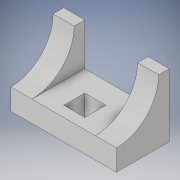
# Autodesk Inventor part: Part2
Saved by Autodesk Inventor 2017 (Build 210142000, 142)
## iProperties
Created: 2016-11-01
Part Number: Part2
Material: Generic
Document SubType Name: Modeling
Designer: s411888
Density: 1 g/cm^3
Appearance: Default
Author: s411888
Autodesk Inventor part; units mm, degrees
ref_plane "YZ Plane" through (0, 0, 0) normal (1, 0, 0) x (0, 1, 0)
ref_plane "XZ Plane" through (0, 0, 0) normal (0, 1, 0) x (-1, 0, 0)
ref_plane "XY Plane" through (0, 0, 0) normal (0, 0, 1) x (1, 0, 0)
sketch "Sketch1" plane through (0, 0, 0) normal (0, 1, 0) x (-1, 0, 0)
  line L0 (35.0198, 16.1328) -> (-28.4802, 16.1328)
  line L1 (-28.4802, 16.1328) -> (-28.4802, -15.6172)
  line L2 (-28.4802, -15.6172) -> (35.0198, -15.6172)
  line L3 (35.0198, -15.6172) -> (35.0198, 16.1328)
  point P0 (0, 0)
  dimension "d0" = 63.5
  dimension "d1" = 31.75
  constraints: 8 end point, 2 parallel, 1 horizontal, 1 perpendicular
  measures "d0" distance of L2.end L1.end
  measures "d1" distance of L0.end L1.end
extrude "Extrusion1" add sketch "Sketch1" along normal blind 38.1
sketch "Sketch2" plane through (0, 38.1, 0) normal (0, 1, 0) x (1, 0, 0)
  line L0 (28.4802, -16.1328) -> (28.4802, 15.6172) projected
  line L1 (15.7802, 15.6172) -> (15.7802, 9.2672)
  line L2 (28.4802, 9.2672) -> (28.4802, 15.6172)
  line L3 (15.7802, 15.6172) -> (-22.3198, 15.6172)
  line L4 (-22.3198, 15.6172) -> (-22.3198, -16.1328)
  line L5 (-22.3198, -16.1328) -> (15.7802, -16.1328)
  line L6 (15.7802, -16.1328) -> (15.7802, 15.6172)
  point P0 (0, 0)
  dimension "d4" = 12.7
  dimension "d5" = 6.35
  dimension "d6" = 38.1
  dimension "d7" = 31.75
  constraints: 12 end point, 3 parallel, 1 horizontal, 1 perpendicular
  measures "d4" distance of L2.start L1.end
  measures "d5" distance of L1.end L1.start
  measures "d6" distance of L5.end L4.end
  measures "d7" distance of L3.end L4.end
extrude "Extrusion2" cut sketch "Sketch2" against normal blind 25.4
sketch "Sketch3" plane through (28.4802, 0, 16.1328) normal (1, 0, 0) x (0, 0, -1)
  line L0 (0, 12.7) -> (0, 38.1) projected
  circle A0 centre (0, 38.1) radius 25.4
  point P0 (16.1328, 0)
  dimension "d10" = 50.8
  constraints: 1 centre point
  measures "d10" diameter of A0
extrude "Extrusion3" cut sketch "Sketch3" against normal blind 76.2
sketch "Sketch4" plane through (0, 12.7, 0) normal (0, 1, 0) x (1, 0, 0)
  line L0 (28.4802, 15.6172) -> (-35.0198, 15.6172) projected
  line L1 (15.8725, 15.6172) -> (3.1725, 15.6172)
  line L2 (15.8725, 2.9172) -> (15.8725, 15.6172)
  line L3 (3.1725, 2.9172) -> (-9.5275, 2.9172)
  line L4 (-9.5275, 2.9172) -> (-9.5275, -9.7828)
  line L5 (-9.5275, -9.7828) -> (3.1725, -9.7828)
  line L6 (3.1725, -9.7828) -> (3.1725, 2.9172)
  point P0 (0, 0)
  dimension "d13" = 12.7
  dimension "d14" = 12.7
  dimension "d15" = 12.7
  dimension "d16" = 12.7
  constraints: 12 end point, 2 horizontal, 2 parallel, 1 perpendicular, 1 point on line
  measures "d13" distance of L2.start L3.start
  measures "d14" distance of L3.start L1.end
  measures "d15" distance of L5.end L4.end
  measures "d16" distance of L4.end L3.end
extrude "Extrusion4" cut sketch "Sketch4" against normal blind 25.4
body "Solid1"
